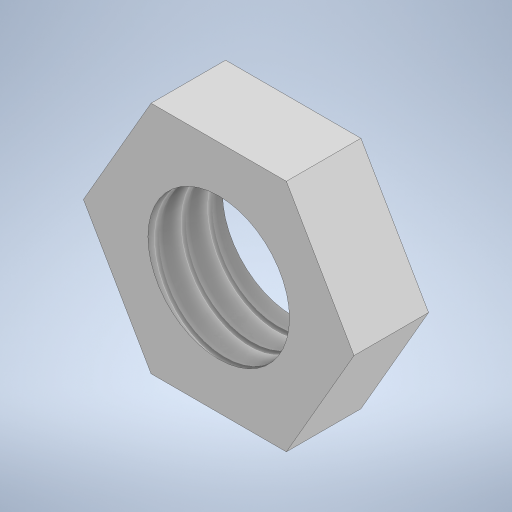
# Autodesk Inventor part: HUDSON-1-89A
Saved by Autodesk Inventor 2024.2 (Build 282272000, 272)
## iProperties
Created: 2024-10-06
Part Number: HUDSON-1-89A
Material: Generic
Document SubType Name: Modeling
Designer: melim
Density: 1 g/cm^3
Appearance: Default
Author: melim
Autodesk Inventor part; units mm, degrees
ref_plane "YZ Plane" through (0, 0, 0) normal (1, 0, 0) x (0, 1, 0)
ref_plane "XZ Plane" through (0, 0, 0) normal (0, 1, 0) x (-1, 0, 0)
ref_plane "XY Plane" through (0, 0, 0) normal (0, 0, 1) x (1, 0, 0)
sketch "Sketch1" plane through (0, 0, 0) normal (0, 0, 1) x (1, 0, 0)
  line L0 (0, 0) -> (0, -16) construction
  line L1 (-3.1754, -13.5) -> (-6.3509, -8)
  line L2 (-6.3509, -8) -> (-3.1754, -2.5)
  line L3 (-3.1754, -2.5) -> (3.1754, -2.5)
  line L4 (3.1754, -2.5) -> (6.3509, -8)
  line L5 (6.3509, -8) -> (3.1754, -13.5)
  line L6 (3.1754, -13.5) -> (-3.1754, -13.5)
  point P0 (0, -8)
  point P1 (0, -2.5)
  point P2 (-4.7631, -5.25)
  dimension "d0" = 11
  constraints: 14 end point, 3 midpoint, 1 point on line, 1 vertical, 13 other
  measures "d0" distance from line of L5 point (-4.763, -5.25)
extrude "Extrusion1" add sketch "Sketch1" along normal blind 3.5
hole "Hole1" at (0, -8, 0) direction (0, 0, 1) diameter 6.647 end through all thread size "M8x1.25" class "6H" standard "ANSI Metric M Profile"
body "Solid1"
